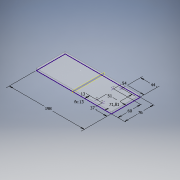
# Autodesk Inventor part: BT703_trajan20_21
Saved by Autodesk Inventor 2022.2 (Build 262287000, 287)
## iProperties
Company: HTBLA Kaindorf
RuleStatus: InUse
Created: 2022-08-21
Part Number: BT703_trajan20_21
Project: Zeichenmaschine_v2
Material: Acryl
Description: Plexitür_200x80
Document SubType Name: Modeling
Designer: trajan20
Density: 1.188 g/cm^3
Appearance: Transparent - farblos
Mass: 89.1974 g
Surface Area: 329.348 cm^2
Volume: 75.082 cm^3
AfterDocNew0: iProperties-Editor_aufrufen
Author: jan
Keywords: 2021
Autodesk Inventor part; units mm, degrees
ref_plane "YZ Plane" through (0, 0, 0) normal (1, 0, 0) x (0, 1, 0)
ref_plane "XZ Plane" through (0, 0, 0) normal (0, 1, 0) x (-1, 0, 0)
ref_plane "XY Plane" through (0, 0, 0) normal (0, 0, 1) x (1, 0, 0)
sketch "Skizze3" plane through (0, 0, 0) normal (0, 0, 1) x (1, 0, 0)
  line L0 (0, 0) -> (-76, 0)
  line L1 (-76, 0) -> (-76, 198)
  line L2 (-76, 198) -> (0, 198)
  line L3 (0, 198) -> (0, 0)
  point P0 (-13, 161)
  point P1 (-13, 147)
  point P2 (-71.81, 154)
  point P3 (-60, 144)
  dimension "d4" = 198
  dimension "d5" = 76
  dimension "d9" = 37
  dimension "d10" = 51
  dimension "d11" = 13
  dimension "d12" = 13
  dimension "d13" = 71.81
  dimension "d14" = 44
  dimension "d15" = 60
  dimension "d16" = 54
  constraints: 8 end point, 2 parallel, 1 horizontal, 1 perpendicular
  measures "d4" distance between parallel lines of L0 L2
  measures "d5" distance between parallel lines of L1 L3
  measures "d9" distance from line of point (-13, 161) L2
  measures "d10" distance from line of point (-13, 147) L2
  measures "d11" distance from line of L3 point (-13, 161)
  measures "d12" distance from line of L3 point (-13, 147)
  measures "d13" distance from line of L3 point (-71.81, 154)
  measures "d14" distance from line of L2 point (-71.81, 154)
  measures "d15" distance from line of L3 point (-60, 144)
  measures "d16" distance from line of point (-60, 144) L2
extrude "Extrusion3" add sketch "Skizze3" along normal blind 5
fillet "Rundung1" radius 2 4 edges at (0, 198, 2.5) (-76, 198, 2.5) (-76, 0, 2.5) (0, 0, 2.5)
ref_plane "Arbeitsebene1" through (-76, 99, 0) normal (0, -1, 0) x (1, 0, 0)
hole "Bohrung1" at (-13, 161, 0) at (-13, 147, 0) at (-60, 144, 0) direction (0, 0, 1) diameter 3.242 end through all thread size "M4x0.7" class "6H" standard "ISO Metric profile"
hole "Bohrung2" at (-71.81, 154, 0) direction (0, 0, 1) diameter 1.567 depth 4.2 tip angle 118 countersink diameter 4.5 countersink angle 90 thread size "M2x0.4" class "6H" standard "ISO Metric profile"
equation "\"d12\" = d11"
